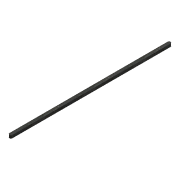
# Autodesk Inventor part: Part3
Saved by Autodesk Inventor 2017 (Build 210142000, 142)
## iProperties
Created: 2019-05-25
Part Number: Part3
Material: Steel
Document SubType Name: Modeling
Designer: Admin
Density: 7.85 g/cm^3
Appearance: Plate
Mass: 437.422 g
Surface Area: 225.843 cm^2
Volume: 55.7226 cm^3
Author: Admin
Autodesk Inventor part; units mm, degrees
ref_plane "YZ Plane" through (0, 0, 0) normal (1, 0, 0) x (0, 1, 0)
ref_plane "XZ Plane" through (0, 0, 0) normal (0, 1, 0) x (-1, 0, 0)
ref_plane "XY Plane" through (0, 0, 0) normal (0, 0, 1) x (1, 0, 0)
sketch "Sketch1" plane through (0, 0, 0) normal (0, 0, 1) x (1, 0, 0)
  line L0 (0, 0) -> (0, 550) construction
  line L1 (5, 0) -> (5, 550)
  line L2 (-5, 550) -> (-5, 0)
  arc A0 (-5, 0) -> (5, 0) centre (0, 0) ccw
  arc A1 (5, 550) -> (-5, 550) centre (0, 550) ccw
  circle A2 centre (0, 0) radius 1
  circle A3 centre (0, 550) radius 1
  point P0 (0, 275)
  dimension "d0" = 550
  dimension "d1" = 10
  dimension "d2" = 2
  dimension "d3" = 2
  constraints: 8 end point, 4 centre point, 4 point on circle, 4 tangent, 2 coincident, 1 midpoint, 1 parallel, 1 vertical
  measures "d0" distance of L0.start L0.end
  measures "d1" diameter of A1
  measures "d2" diameter of A2
  measures "d3" diameter of A3
extrude "Extrusion1" add sketch "Sketch1" along normal blind 10
body "Solid1"
